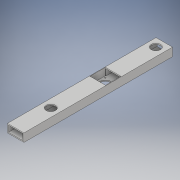
# Autodesk Inventor part: 1x2 arm
Saved by Autodesk Inventor 2018 (Build 220112000, 112)
## iProperties
Created: 2018-01-20
Part Number: 1x2 arm
Material: Generic
Document SubType Name: Modeling
Designer: Apple
Density: 1 g/cm^3
Appearance: Default
Author: Apple
Autodesk Inventor part; units mm, degrees
ref_plane "YZ Plane" through (0, 0, 0) normal (1, 0, 0) x (0, 1, 0)
ref_plane "XZ Plane" through (0, 0, 0) normal (0, 1, 0) x (-1, 0, 0)
ref_plane "XY Plane" through (0, 0, 0) normal (0, 0, 1) x (1, 0, 0)
sketch "Sketch1" plane through (0, 0, 0) normal (0, 0, 1) x (1, 0, 0)
  line L0 (-59.9006, 6.3636) -> (-15.4506, 6.3636)
  line L1 (-15.4506, 6.3636) -> (-15.4506, -12.6864)
  line L2 (-15.4506, -12.6864) -> (-59.9006, -12.6864)
  line L3 (-59.9006, -12.6864) -> (-59.9006, 6.3636)
  line L4 (-63.0756, 9.5386) -> (-12.2756, 9.5386)
  line L5 (-12.2756, 9.5386) -> (-12.2756, -15.8614)
  line L6 (-12.2756, -15.8614) -> (-63.0756, -15.8614)
  line L7 (-63.0756, -15.8614) -> (-63.0756, 9.5386)
  point P0 (0, 0)
  dimension "d2" = 3.175
  dimension "d5" = 50.8
  dimension "d6" = 25.4
  constraints: 16 end point, 4 parallel, 2 perpendicular, 1 horizontal, 3 other
  measures "d2" distance between parallel lines of L3 L7
  measures "d5" distance between parallel lines of L5 L7
  measures "d6" distance of L6.end L4.start
extrude "Extrusion1" add sketch "Sketch1" along normal blind 457.2
sketch "Sketch4" plane through (-63.0756, 9.5386, 0) normal (0, 1, 0) x (1, 0, 0)
  circle A0 centre (24.9171, -25.4) radius 14.2621
  line L0 (0, 0) -> (50.8, 0) projected
  point P0 (63.0756, 0)
  dimension "d13" = 28.5242
  dimension "d14" = 25.4
  constraints: 1 centre point
  measures "d13" diameter of A0
  measures "d14" distance from line of L0 A0.centre
extrude "Extrusion4" cut sketch "Sketch4" against normal through all
sketch "Sketch2" plane through (-63.0756, 9.5386, 0) normal (0, 1, 0) x (1, 0, 0)
  line L0 (1.5875, -157.1625) -> (49.2125, -157.1625)
  line L1 (49.2125, -157.1625) -> (49.2125, -204.7875)
  line L2 (49.2125, -204.7875) -> (1.5875, -204.7875)
  line L3 (1.5875, -204.7875) -> (1.5875, -157.1625)
  line L4 (50.8, -457.2) -> (0, -457.2) projected
  circle A0 centre (24.9171, -25.4) radius 14.2621 projected
  line L5 (0, 0) -> (50.8, 0) projected
  point P0 (63.0756, 0)
  point P1 (25.4, -204.7875)
  point P2 (25.4, -457.2)
  dimension "d7" = 47.625
  dimension "d8" = 47.625
  dimension "d24" = 157.1625
  constraints: 8 end point, 2 midpoint, 2 parallel, 1 horizontal, 1 perpendicular, 1 vertical alignment
  measures "d7" distance of L0.start L0.end
  measures "d8" distance of L0.end L1.end
  measures "d24" distance between parallel lines of L0 L5
extrude "Extrusion2" cut sketch "Sketch2" against normal up to surface (22.225 mm away) contours L0 L1 L2 L3
sketch "Sketch9" plane through (-59.9006, -12.6864, 0) normal (0, 1, 0) x (1, 0, 0)
  circle A0 centre (21.7421, -180.975) radius 16.7645
  line L0 (-1.5875, -204.7875) -> (-1.5875, -157.1625) projected
  circle A1 centre (21.7421, -25.4) radius 14.2621 projected
  circle A2 centre (3.4541, -199.263) radius 1.7
  circle A3 centre (40.0301, -199.263) radius 1.7
  circle A4 centre (40.0301, -162.687) radius 1.7
  circle A5 centre (3.4541, -162.687) radius 1.7
  point P0 (59.9006, 0)
  point P1 (-1.5875, -180.975)
  dimension "d34" = 18.288
  dimension "d35" = 18.288
  dimension "d38" = 360
  constraints: 5 centre point, 1 horizontal alignment, 1 midpoint, 1 vertical alignment, 9 other
  measures "d34" horizontal distance of A2.centre A0.centre
  measures "d35" horizontal distance of A2.centre A0.centre
extrude "Extrusion8" cut sketch "Sketch9" against normal through all contours A0 | A2 | A3 | A4 | A5
sketch "Sketch10" plane through (-63.0756, 9.5386, 0) normal (0, 1, 0) x (1, 0, 0)
  circle A0 centre (25.4, -349.25) radius 14.2875
  line L0 (50.8, -457.2) -> (0, -457.2) projected
  line L1 (0, 0) -> (50.8, 0) projected
  point P0 (63.0756, 0)
  point P1 (25.4, -457.2)
  dimension "d42" = 28.575
  dimension "d43" = 349.25
  constraints: 1 centre point, 1 midpoint, 1 vertical alignment
  measures "d42" diameter of A0
  measures "d43" distance from line of L1 A0.centre
extrude "Extrusion9" cut sketch "Sketch10" against normal through all
equation "\"d8\" = d7"
equation "\"d35\" = d34"
body "Solid1"
